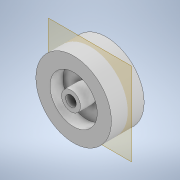
# Autodesk Inventor part: wheel
Saved by Autodesk Inventor 2022 (Build 260153000, 153)
## iProperties
Created: 2022-04-20
Part Number: wheel
Material: Generic
Document SubType Name: Modeling
Designer: Yazawa
Density: 1 g/cm^3
Appearance: Default
Author: Yazawa
Autodesk Inventor part; units mm, degrees
ref_plane "YZ Plane" through (0, 0, 0) normal (1, 0, 0) x (0, 1, 0)
ref_plane "XZ Plane" through (0, 0, 0) normal (0, 1, 0) x (-1, 0, 0)
ref_plane "XY Plane" through (0, 0, 0) normal (0, 0, 1) x (1, 0, 0)
sketch "スケッチ1" plane through (0, 0, 0) normal (0, 0, 1) x (1, 0, 0)
  circle A0 centre (0, 0) radius 16
  dimension "d0" = 32
  constraints: 1 centre point, 1 coincident
  measures "d0" diameter of A0
extrude "押し出し1" add sketch "スケッチ1" along normal blind 13.88
sketch "スケッチ2" plane through (0, 0, 13.88) normal (0, 0, 1) x (1, 0, 0)
  circle A0 centre (0, 0) radius 16 projected
  circle A1 centre (0, 0) radius 10
  circle A2 centre (0, 0) radius 4
  dimension "d3" = 6
  dimension "d4" = 6
  constraints: 2 centre point
  measures "d3" radial gap between concentric circles of A0 A1
  measures "d4" radial gap between concentric circles of A1 A2
extrude "押し出し2" cut sketch "スケッチ2" against normal blind 5.5 contours A1
ref_plane "作業平面1" through (0, 0, 6.94) normal (0, 0, 1) x (1, 0, 0)
mirror "ミラー1" about plane through (0, 0, 6.94) normal (0, 0, 1) of "押し出し2"
sketch "スケッチ3" plane through (0, 0, 13.88) normal (0, 0, 1) x (1, 0, 0)
  point P0 (0, 0)
  point P1 (0, 0)
  constraints: 1 coincident
hole "穴1" at (0, 0, 13.88) direction (0, 0, -1) diameter 4.5 depth 13.88
sketch "スケッチ4" plane through (0, 0, 13.88) normal (0, 0, 1) x (1, 0, 0)
  circle A0 centre (0, 0) radius 2.25 projected
  circle A1 centre (0, 0) radius 4 projected
extrude "押し出し3" add sketch "スケッチ4" along normal blind 1.11
mirror "ミラー2" about plane through (0, 0, 6.94) normal (0, 0, 1) of "押し出し3"
